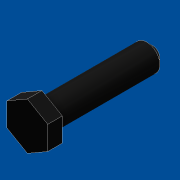
# Autodesk Inventor part: perno_38
Saved by Autodesk Inventor 2016 (Build 200138000, 138)
## iProperties
Created: 2017-05-13
Part Number: perno_38
Material: Generic
Document SubType Name: Modeling
Designer: Gian
Density: 1 g/cm^3
Appearance: Default
Author: Gian
Autodesk Inventor part; units mm, degrees
ref_plane "YZ Plane" through (0, 0, 0) normal (1, 0, 0) x (0, 1, 0)
ref_plane "XZ Plane" through (0, 0, 0) normal (0, 1, 0) x (-1, 0, 0)
ref_plane "XY Plane" through (0, 0, 0) normal (0, 0, 1) x (1, 0, 0)
sketch "Sketch1" plane through (0, 0, 0) normal (0, 1, 0) x (-1, 0, 0)
  line L0 (7.5201, 21.3562) -> (14.5201, 17.3147)
  line L1 (14.5201, 17.3147) -> (14.5201, 9.2318)
  line L2 (14.5201, 9.2318) -> (7.5201, 5.1904)
  line L3 (7.5201, 5.1904) -> (0.5201, 9.2318)
  line L4 (0.5201, 9.2318) -> (0.5201, 17.3147)
  line L5 (0.5201, 17.3147) -> (7.5201, 21.3562)
  point P0 (7.5201, 13.2733)
  dimension "d0" = 14
  constraints: 12 end point, 1 vertical, 13 other
  measures "d0" distance between parallel lines of L4 L1
extrude "Extrusion1" add sketch "Sketch1" along normal blind 5
sketch "Sketch2" plane through (0, 5, 0) normal (0, 1, 0) x (1, 0, 0)
  line L0 (-14.5201, -17.3147) -> (-7.5201, -21.3562) projected
  line L1 (-7.5201, -21.3562) -> (-0.5201, -17.3147) projected
  line L2 (-0.5201, -17.3147) -> (-0.5201, -9.2318) projected
  line L3 (-0.5201, -9.2318) -> (-7.5201, -5.1904) projected
  line L4 (-7.5201, -5.1904) -> (-14.5201, -9.2318) projected
  line L5 (-14.5201, -9.2318) -> (-14.5201, -17.3147) projected
  line L6 (-14.5201, -13.2733) -> (-0.5201, -13.2733) construction
  circle A0 centre (-7.5201, -13.2733) radius 4.5
  dimension "d3" = 9
  constraints: 3 midpoint, 2 end point, 1 centre point
  measures "d3" diameter of A0
extrude "Extrusion2" add sketch "Sketch2" along normal blind 38 contours A0
chamfer "Chamfer1" distance 2 angle 45 1 edges at (-12.0201, 43, 13.2733)
body "Solid1"
